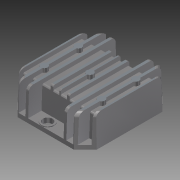
# Autodesk Inventor part: CS_Converter_CLL25-24S05
Saved by Autodesk Inventor 2013 (Build 170138000, 138)
## iProperties
Category: Control Systems
Company: Autodesk Inc.
Created: 2012-11-30
Part Number: CS_Converter_CLL25-24S05
Material: Steel, Galvanized
Document SubType Name: Modeling
Designer: Autodesk Inc.
Density: 7.85 g/cm^3
Mass: 481.89 g
Surface Area: 175.529 cm^2
Volume: 61.3872 cm^3
Author: Autodesk Inc.
Autodesk Inventor part; units mm, degrees
sketch "Sketch1" plane through (0, 0, 0) normal (0, 0, 1) x (1, 0, 0)
  line L0 (-8.505175, 8.505175) -> (0, 0)
  line L1 (0, 0) -> (48.98965, 0)
  line L2 (48.98965, 0) -> (57.494825, 8.505175)
  line L3 (57.494825, 8.505175) -> (57.494825, 50.494825)
  line L4 (57.494825, 50.494825) -> (48.98965, 59)
  line L5 (0, 59) -> (48.98965, 59)
  line L6 (0, 59) -> (-8.505175, 50.494825)
  line L7 (-8.505175, 8.505175) -> (-8.505175, 50.494825)
  circle A0 centre (-3.505175, 26) radius 3.5
  circle A1 centre (52.456027, 26) radius 3.5
  point P0 (24.475426, 0)
  constraints: 16 end point, 2 centre point
sketch "Sketch1 outline for Extrusion1" plane through (0, 0, 0) normal (0, 0, 1) x (1, 0, 0)
  line L0 (-8.505175, 50.494825) -> (-8.505175, 8.505175)
  line L1 (0, 59) -> (-8.505175, 50.494825)
  line L2 (48.98965, 59) -> (0, 59)
  line L3 (57.494825, 50.494825) -> (48.98965, 59)
  line L4 (57.494825, 8.505175) -> (57.494825, 50.494825)
  line L5 (48.98965, 0) -> (57.494825, 8.505175)
  line L6 (0, 0) -> (48.98965, 0)
  line L7 (-8.505175, 8.505175) -> (0, 0)
extrude "Extrusion1" add sketch "Sketch1 outline for Extrusion1" against normal blind 23.0124 draft -2
sketch "Sketch4" plane through (0, 0, -23.0124) normal (0, 0, -1) x (-1, 0, 0)
  line L0 (-0.332866, 0.803611) -> (-48.656784, 0.803611)
  line L1 (-56.221336, 44.750433) -> (-56.221336, 42.750433)
  line L2 (-56.221336, 42.750433) -> (8.172308, 42.750433)
  line L3 (8.172308, 42.750433) -> (8.172308, 44.750433)
  line L4 (8.172308, 44.750433) -> (-56.221336, 44.750433)
  line L5 (-63.041798, 16.272211) -> (14.051617, 16.272211)
  line L6 (14.051617, 14.265611) -> (-63.041798, 14.265611)
  line L7 (-56.221336, 42.750433) -> (-56.221336, 44.750433)
  line L8 (-56.221336, 44.750433) -> (8.172308, 44.750433)
  line L9 (8.172308, 44.750433) -> (8.172308, 42.750433)
  line L10 (8.172308, 42.750433) -> (-56.221336, 42.750433)
  line L11 (0.863956, 57.000433) -> (-48.912984, 57.000433)
  line L12 (-48.912984, 57.000433) -> (-47.716161, 58.197255)
  line L13 (-47.716161, 58.197255) -> (-0.332866, 58.197255)
  line L14 (-0.332866, 58.197255) -> (0.863956, 57.000433)
  line L15 (-54.037984, 51.875433) -> (5.988956, 51.875433)
  line L16 (5.988956, 51.875433) -> (7.988956, 49.875433)
  line L17 (7.988956, 49.875433) -> (-56.037984, 49.875433)
  line L18 (-56.037984, 49.875433) -> (-54.037984, 51.875433)
  line L19 (14.051617, 7.128211) -> (-63.041798, 7.128211)
  line L20 (-63.041798, 1.997411) -> (14.051617, 1.997411)
  line L21 (14.051617, 0.803611) -> (-63.041798, 0.803611)
  line L22 (-46.221336, 37.625433) -> (-1.827692, 37.625433)
  line L23 (-1.827692, 37.625433) -> (-1.827692, 35.625433)
  line L24 (-1.827692, 35.625433) -> (-46.221336, 35.625433)
  line L25 (-46.221336, 35.625433) -> (-46.221336, 37.625433)
  line L26 (-46.221336, 30.998233) -> (-1.827692, 30.998233)
  line L27 (-1.827692, 30.998233) -> (-1.827692, 28.998233)
  line L28 (14.051617, 28.998233) -> (-63.041798, 28.998233)
  line L29 (-46.221336, 28.998233) -> (-46.221336, 30.998233)
  line L30 (-63.041798, 24.375433) -> (14.051617, 24.375433)
  line L31 (-1.827692, 24.375433) -> (-1.827692, 22.375433)
  line L32 (14.051617, 22.375433) -> (-63.041798, 22.375433)
  line L33 (-46.221336, 22.375433) -> (-46.221336, 24.375433)
  line L34 (14.051617, -5.546389) -> (-63.041798, -5.546389)
  line L35 (-63.041798, 62.372027) -> (14.051617, 62.372027)
  line L36 (14.051617, 9.134811) -> (-63.041798, 9.134811)
  line L37 (-63.041798, 9.134811) -> (-63.041798, 14.265611)
  line L38 (-63.041798, -5.546389) -> (-63.041798, 0.803611)
  line L39 (-63.041798, 1.997411) -> (-63.041798, 7.128211)
  line L40 (14.051617, 0.803611) -> (14.051617, -5.546389)
  line L41 (14.051617, 7.128211) -> (14.051617, 1.997411)
  line L42 (14.051617, 14.265611) -> (14.051617, 9.134811)
  line L43 (-63.041798, 16.272211) -> (-63.041798, 22.375433)
  line L44 (-63.041798, 24.375433) -> (-63.041798, 62.372027)
  line L45 (14.051617, 62.372027) -> (14.051617, 24.375433)
  line L46 (14.051617, 22.375433) -> (14.051617, 16.272211)
  point P0 (0, 0)
  point P1 (-24.043913, 59.000433)
  dimension "d6" = 6.35
  dimension "d7" = 1.1938
  dimension "d8" = 5.1308
  dimension "d9" = 2.0066
  dimension "d10" = 5.1308
  dimension "d11" = 2.0066
  dimension "d14" = 6.10322
  dimension "d16" = 4.6228
  constraints: 92 end point, 27 parallel, 8 point on line, 5 perpendicular, 2 horizontal, 1 collinear
  measures "d6" distance between parallel lines of L34 L0
  measures "d7" distance between parallel lines of L20 L21
  measures "d8" distance between parallel lines of L19 L20
  measures "d9" distance between parallel lines of L36 L19
  measures "d10" distance between parallel lines of L6 L36
  measures "d11" distance between parallel lines of L5 L6
  measures "d14" distance between parallel lines of L32 L5
  measures "d16" distance between parallel lines of L28 L30
extrude "Extrusion3" cut sketch "Sketch4" against normal blind 19.9898 contours L43 L32 L46 L5 | L30 L44 L28 L45 | L42 L36 L37 L6 | L41 L20 L39 L19
ref_plane "Work Plane1" through (-8.505175, 29.5, 0) normal (0, -1, 0) x (1, 0, 0)
mirror "Mirror1" about plane through (-8.505175, 29.5, 0) normal (0, -1, 0) of "Extrusion3"
ref_plane "Work Plane2" through (48.98965, 59, 0) normal (0, 1, 0) x (-1, 0, 0)
sketch "Sketch5" plane through (48.98965, 59, 0) normal (0, 1, 0) x (-1, 0, 0)
  line L0 (50.837789, -3.0226) -> (55.968589, -3.0226)
  line L1 (-6.978938, -3.0226) -> (-1.848138, -3.0226)
  line L2 (50.837789, -3.0226) -> (-1.848138, -3.0226)
  line L3 (1.599587, -3.0226) -> (-6.915475, -3.0226)
  line L4 (55.905126, -3.0226) -> (47.390063, -3.0226)
  line L5 (1.599587, -3.0226) -> (47.390063, -3.0226)
  line L6 (2.193241, -20.0226) -> (1.599587, -3.0226)
  line L7 (46.79641, -20.0226) -> (2.193241, -20.0226)
  line L8 (47.390063, -3.0226) -> (46.79641, -20.0226)
  point P0 (48.98965, 0)
  point P1 (24.494825, -3.0226)
  point P2 (24.494825, -3.0226)
  constraints: 12 end point, 2 midpoint
extrude "Extrusion4" add sketch "Sketch5" along normal up to surface (55.005179 mm away) from surface at -57.002589
sketch "Sketch7" plane through (-7.701564, 22.375433, -23.0124) normal (0, -1, 0) x (1, 0, 0)
  line L0 (9.301152, 19.9898) -> (-0.698059, 19.9898)
  line L1 (0, 0) -> (-0.698059, 19.9898)
  line L2 (64.392779, 0) -> (0, 0)
  line L3 (9.301152, 19.9898) -> (9.999211, 0)
  point P0 (7.701564, 23.0124)
  constraints: 2 end point, 1 parallel, 1 point on line
extrude "Extrusion5" cut sketch "Sketch7" against normal up to surface (20.352356 mm away)
sketch "Sketch8" plane through (2.297647, 22.375433, -23.0124) normal (0, -1, 0) x (1, 0, 0)
  line L0 (54.393568, 0) -> (0, 0)
  line L1 (55.091627, 19.9898) -> (54.393568, 0)
  line L2 (55.091627, 19.9898) -> (45.092416, 19.9898)
  line L3 (45.092416, 19.9898) -> (44.498763, 2.9898)
  line L4 (45.092416, 19.9898) -> (44.394357, 0)
  point P0 (-2.297647, 23.0124)
  constraints: 2 end point, 1 collinear, 1 point on line
extrude "Extrusion6" cut sketch "Sketch8" against normal up to surface (20.352356 mm away)
extrude "Extrusion7" cut sketch "Sketch1" against normal up to surface (3.0226 mm away) contours A0 | A1
fillet "Fillet1" radius 3.175 12 edges at (-0.264, 1.4005, -23.0124) (-6.8466, 7.9831, -23.0124) (-7.7016, 15.2689, -23.0124) (-7.7016, 43.7311, -23.0124) (-6.8466, 51.0169, -23.0124) (-0.264, 57.5995, -23.0124) (49.2537, 57.5995, -23.0124) (55.8363, 51.0169, -23.0124) (56.6912, 43.7311, -23.0124) (56.6912, 15.2689, -23.0124) (55.8363, 7.9831, -23.0124) (49.2537, 1.4005, -23.0124)
fillet "Fillet2" radius 1.27 6 edges at (2.2976, 23.3754, -23.0124) (2.2976, 29.5, -23.0124) (2.2976, 35.6246, -23.0124) (46.692, 23.3754, -23.0124) (46.692, 29.5, -23.0124) (46.692, 35.6246, -23.0124)
fillet "Fillet3" radius 1.27 16 edges at (2.1932, 4.5628, -20.0226) (2.1932, 11.7002, -20.0226) (2.1932, 19.3238, -20.0226) (2.1932, 26.6868, -20.0226) (2.1932, 32.3132, -20.0226) (2.1932, 39.6762, -20.0226) (2.1932, 47.2998, -20.0226) (2.1932, 54.4372, -20.0226) (46.7964, 4.5628, -20.0226) (46.7964, 11.7002, -20.0226) (46.7964, 19.3238, -20.0226) (46.7964, 26.6868, -20.0226) (46.7964, 32.3132, -20.0226) (46.7964, 39.6762, -20.0226) (46.7964, 47.2998, -20.0226) (46.7964, 54.4372, -20.0226)
sketch "Sketch9" plane through (0, 0, -23.0124) normal (0, 0, -1) x (-1, 0, 0)
  line L0 (-50.645318, 7.128211) -> (-52.651918, 9.134811)
  line L1 (-50.645318, 7.128211) -> (1.655667, 7.128211)
  circle A0 centre (-37.194825, 8.131511) radius 2.54
  circle A1 centre (-11.794825, 8.131511) radius 2.54
  line L2 (-45.465579, 28.998233) -> (-45.465579, 30.001767)
  line L3 (-45.465579, 28.998233) -> (-3.524071, 28.998233)
  line L4 (-3.524071, 30.001767) -> (-3.524071, 28.998233)
  line L5 (-3.524071, 30.001767) -> (-45.465579, 30.001767)
  circle A2 centre (-24.494825, 29.5) radius 2.54
  line L6 (-37.194825, 8.131511) -> (-11.794825, 8.131511) construction
  point P0 (0, 0)
  point P1 (-45.465579, 29.5)
  point P2 (-51.648618, 8.131511)
  point P3 (-3.524071, 29.5)
  point P4 (-24.494825, 30.001767)
  point P5 (-24.494825, 8.131511)
  dimension "d29" = 5.08
  dimension "d32" = 25.4
  constraints: 5 midpoint, 4 horizontal alignment, 3 centre point, 2 end point, 2 equal radius, 2 vertical alignment, 1 parallel
  measures "d29" diameter of A0
  measures "d32" distance of L6.end L6.start
extrude "Extrusion8" add sketch "Sketch9" against normal up to surface (2.9898 mm away) contours A0 L1 | L1 A0 | A1 L1 | L1 A1 | A2 L5 L3 | L3 A2 | A2 L5
ref_plane "Work Plane3" through (3.419665, 29.5, -20.0226) normal (0, 1, 0) x (1, 0, 0)
mirror "Mirror2" about plane through (3.419665, 29.5, -20.0226) normal (0, 1, 0) of "Extrusion8"
sketch "Sketch10" plane through (0, 0, -3.0226) normal (0, 0, -1) x (-1, 0, 0)
  circle A0 centre (3.505175, 26) radius 3.5
  circle A1 centre (-52.456027, 26) radius 3.5
  circle A2 centre (-52.456027, 26) radius 4.7625
  circle A3 centre (3.505175, 26) radius 4.7625
  point P0 (0, 0)
  dimension "d35" = 9.525
  constraints: 2 centre point, 1 equal radius
  measures "d35" diameter of A2
extrude "Extrusion9" add sketch "Sketch10" along normal blind 0.508 draft -2
equation "\"d6\" = d5"
equation "\"d11\" = d9"
equation "\"d5\" = d4"
equation "\"d4\" = 6.35"
body "Solid1"
